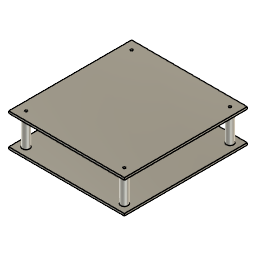
base_colonnine_integrate_dadi_M3_senza_passacavi (Autodesk Fusion 360 design; units mm, degrees)
part number: 2026-07-13-14-09-58-204
part number: 2026-07-13-14-09-58-519
part number: 2026-07-13-14-09-58-558
Autodesk Fusion 360 part; units mm, degrees
sketch "Schizzo1" plane through (0, 0, 0) normal (0, 0, 1) x (1, 0, 0) in component "01_Piano_inferiore_con_colonnine_M3"
  line L0 (-80, -85) -> (80, -85)
  line L1 (80, -85) -> (80, 85)
  line L2 (80, 85) -> (-80, 85)
  line L3 (-80, 85) -> (-80, -85)
extrude "Estrusione_Piano_inferiore" add sketch "Schizzo1" along normal blind 3 makes body 1 in component "01_Piano_inferiore_con_colonnine_M3"
ref_plane "Piano di lavoro1" through (0, 0, 43) normal (0, 0, 1) x (1, 0, 0) in component "02_Piano_superiore"
sketch "Schizzo1 (2)" plane through (0, 0, 43) normal (0, 0, 1) x (1, 0, 0) in component "02_Piano_superiore"
  line L0 (-80, -85) -> (80, -85)
  line L1 (80, -85) -> (80, 85)
  line L2 (80, 85) -> (-80, 85)
  line L3 (-80, 85) -> (-80, -85)
extrude "Estrusione_Piano_superiore" add sketch "Schizzo1 (2)" along normal blind 3 separate body makes body 2 in component "02_Piano_superiore"
ref_plane "Piano di lavoro1" through (0, 0, 3) normal (0, 0, 1) x (1, 0, 0) in component "01_Piano_inferiore_con_colonnine_M3"
ref_plane "Piano di lavoro2" through (0, 0, 40.4) normal (0, 0, 1) x (1, 0, 0) in component "01_Piano_inferiore_con_colonnine_M3"
sketch "Schizzo2" plane through (0, 0, 43) normal (0, 0, 1) x (1, 0, 0) in component "02_Piano_superiore"
  circle A0 centre (-68, -73) radius 1.6
extrude "Foro_M3_superiore_01" cut sketch "Schizzo2" along normal blind 3 bodies 2 in component "02_Piano_superiore"
sketch "Schizzo2 (2)" plane through (0, 0, 3) normal (0, 0, 1) x (1, 0, 0) in component "01_Piano_inferiore_con_colonnine_M3"
  circle A0 centre (-68, -73) radius 5
extrude "Estrusione_Colonnina_M3_01" add sketch "Schizzo2 (2)" along normal blind 40 bodies 1 in component "01_Piano_inferiore_con_colonnine_M3"
sketch "Schizzo3" plane through (0, 0, 0) normal (0, 0, 1) x (1, 0, 0) in component "01_Piano_inferiore_con_colonnine_M3"
  circle A0 centre (-68, -73) radius 1.6
extrude "Foro_passante_M3_colonnina_01" cut sketch "Schizzo3" along normal blind 43 bodies 1 in component "01_Piano_inferiore_con_colonnine_M3"
sketch "Schizzo4" plane through (0, 0, 40.4) normal (0, 0, 1) x (1, 0, 0) in component "01_Piano_inferiore_con_colonnine_M3"
  line L0 (-65.1, -71.3257) -> (-68, -69.6514)
  line L1 (-68, -69.6514) -> (-70.9, -71.3257)
  line L2 (-70.9, -71.3257) -> (-70.9, -74.6743)
  line L3 (-70.9, -74.6743) -> (-68, -76.3486)
  line L4 (-68, -76.3486) -> (-65.1, -74.6743)
  line L5 (-65.1, -74.6743) -> (-65.1, -71.3257)
extrude "Sede_dado_M3_01" cut sketch "Schizzo4" along normal blind 2.6 bodies 1 in component "01_Piano_inferiore_con_colonnine_M3"
sketch "Schizzo3 (2)" plane through (0, 0, 43) normal (0, 0, 1) x (1, 0, 0) in component "02_Piano_superiore"
  circle A0 centre (68, -73) radius 1.6
extrude "Foro_M3_superiore_02" cut sketch "Schizzo3 (2)" along normal blind 3 bodies 2 in component "02_Piano_superiore"
sketch "Schizzo5" plane through (0, 0, 3) normal (0, 0, 1) x (1, 0, 0) in component "01_Piano_inferiore_con_colonnine_M3"
  circle A0 centre (68, -73) radius 5
extrude "Estrusione_Colonnina_M3_02" add sketch "Schizzo5" along normal blind 40 bodies 1 in component "01_Piano_inferiore_con_colonnine_M3"
sketch "Schizzo6" plane through (0, 0, 0) normal (0, 0, 1) x (1, 0, 0) in component "01_Piano_inferiore_con_colonnine_M3"
  circle A0 centre (68, -73) radius 1.6
extrude "Foro_passante_M3_colonnina_02" cut sketch "Schizzo6" along normal blind 43 bodies 1 in component "01_Piano_inferiore_con_colonnine_M3"
sketch "Schizzo7" plane through (0, 0, 40.4) normal (0, 0, 1) x (1, 0, 0) in component "01_Piano_inferiore_con_colonnine_M3"
  line L0 (70.9, -71.3257) -> (68, -69.6514)
  line L1 (68, -69.6514) -> (65.1, -71.3257)
  line L2 (65.1, -71.3257) -> (65.1, -74.6743)
  line L3 (65.1, -74.6743) -> (68, -76.3486)
  line L4 (68, -76.3486) -> (70.9, -74.6743)
  line L5 (70.9, -74.6743) -> (70.9, -71.3257)
extrude "Sede_dado_M3_02" cut sketch "Schizzo7" along normal blind 2.6 bodies 1 in component "01_Piano_inferiore_con_colonnine_M3"
sketch "Schizzo4 (2)" plane through (0, 0, 43) normal (0, 0, 1) x (1, 0, 0) in component "02_Piano_superiore"
  circle A0 centre (68, 73) radius 1.6
extrude "Foro_M3_superiore_03" cut sketch "Schizzo4 (2)" along normal blind 3 bodies 2 in component "02_Piano_superiore"
sketch "Schizzo8" plane through (0, 0, 3) normal (0, 0, 1) x (1, 0, 0) in component "01_Piano_inferiore_con_colonnine_M3"
  circle A0 centre (68, 73) radius 5
extrude "Estrusione_Colonnina_M3_03" add sketch "Schizzo8" along normal blind 40 bodies 1 in component "01_Piano_inferiore_con_colonnine_M3"
sketch "Schizzo9" plane through (0, 0, 0) normal (0, 0, 1) x (1, 0, 0) in component "01_Piano_inferiore_con_colonnine_M3"
  circle A0 centre (68, 73) radius 1.6
extrude "Foro_passante_M3_colonnina_03" cut sketch "Schizzo9" along normal blind 43 bodies 1 in component "01_Piano_inferiore_con_colonnine_M3"
sketch "Schizzo10" plane through (0, 0, 40.4) normal (0, 0, 1) x (1, 0, 0) in component "01_Piano_inferiore_con_colonnine_M3"
  line L0 (70.9, 74.6743) -> (68, 76.3486)
  line L1 (68, 76.3486) -> (65.1, 74.6743)
  line L2 (65.1, 74.6743) -> (65.1, 71.3257)
  line L3 (65.1, 71.3257) -> (68, 69.6514)
  line L4 (68, 69.6514) -> (70.9, 71.3257)
  line L5 (70.9, 71.3257) -> (70.9, 74.6743)
extrude "Sede_dado_M3_03" cut sketch "Schizzo10" along normal blind 2.6 bodies 1 in component "01_Piano_inferiore_con_colonnine_M3"
sketch "Schizzo5 (2)" plane through (0, 0, 43) normal (0, 0, 1) x (1, 0, 0) in component "02_Piano_superiore"
  circle A0 centre (-68, 73) radius 1.6
extrude "Foro_M3_superiore_04" cut sketch "Schizzo5 (2)" along normal blind 3 bodies 2 in component "02_Piano_superiore"
sketch "Schizzo11" plane through (0, 0, 3) normal (0, 0, 1) x (1, 0, 0) in component "01_Piano_inferiore_con_colonnine_M3"
  circle A0 centre (-68, 73) radius 5
extrude "Estrusione_Colonnina_M3_04" add sketch "Schizzo11" along normal blind 40 bodies 1 in component "01_Piano_inferiore_con_colonnine_M3"
sketch "Schizzo12" plane through (0, 0, 0) normal (0, 0, 1) x (1, 0, 0) in component "01_Piano_inferiore_con_colonnine_M3"
  circle A0 centre (-68, 73) radius 1.6
extrude "Foro_passante_M3_colonnina_04" cut sketch "Schizzo12" along normal blind 43 bodies 1 in component "01_Piano_inferiore_con_colonnine_M3"
sketch "Schizzo13" plane through (0, 0, 40.4) normal (0, 0, 1) x (1, 0, 0) in component "01_Piano_inferiore_con_colonnine_M3"
  line L0 (-65.1, 74.6743) -> (-68, 76.3486)
  line L1 (-68, 76.3486) -> (-70.9, 74.6743)
  line L2 (-70.9, 74.6743) -> (-70.9, 71.3257)
  line L3 (-70.9, 71.3257) -> (-68, 69.6514)
  line L4 (-68, 69.6514) -> (-65.1, 71.3257)
  line L5 (-65.1, 71.3257) -> (-65.1, 74.6743)
extrude "Sede_dado_M3_04" cut sketch "Schizzo13" along normal blind 2.6 bodies 1 in component "01_Piano_inferiore_con_colonnine_M3"
component "01_Piano_inferiore_con_colonnine_M3" placed x (1, 0, 0) y (0, 1, 0) z (0, 0, 1) at (0, 0, 0)
component "02_Piano_superiore" placed x (1, 0, 0) y (0, 1, 0) z (0, 0, 1) at (0, 0, 0)
equation "piano_inf_lunghezza = 170.0 mm" comment "Piano inferiore"
equation "piano_inf_larghezza = 160.0 mm" comment "Piano inferiore"
equation "piano_inf_spessore = 3.0 mm" comment "Piano inferiore"
equation "d4 = piano_inf_spessore"
equation "distanza_piani = 40.0 mm" comment "Luce libera fra i piani"
equation "piano_sup_lunghezza = 170.0 mm" comment "Piano superiore"
equation "piano_sup_larghezza = 160.0 mm" comment "Piano superiore"
equation "piano_sup_spessore = 3.0 mm" comment "Piano superiore"
equation "colonnina_diametro = 10.0 mm" comment "Colonnine base"
equation "foro_vite_M3 = 3.2 mm" comment "Gioco vite M3"
equation "colonnina_offset_bordo = 12.0 mm" comment "Centro colonnina dal bordo"
equation "dado_M3_chiave = 5.8 mm" comment "Sede esagonale dado M3"
equation "dado_M3_profondita = 2.6 mm" comment "Profondita sede dado M3"
equation "d15 = piano_inf_spessore + distanza_piani"
equation "d16 = piano_sup_spessore"
equation "d18 = piano_inf_spessore"
equation "d19 = piano_inf_spessore + distanza_piani - dado_M3_profondita"
equation "d20 = piano_sup_spessore"
equation "d22 = distanza_piani"
equation "d24 = piano_inf_spessore + distanza_piani"
equation "d26 = dado_M3_profondita"
equation "d28 = piano_sup_spessore"
equation "d30 = distanza_piani"
equation "d32 = piano_inf_spessore + distanza_piani"
equation "d34 = dado_M3_profondita"
equation "d36 = piano_sup_spessore"
equation "d38 = distanza_piani"
equation "d40 = piano_inf_spessore + distanza_piani"
equation "d42 = dado_M3_profondita"
equation "d44 = piano_sup_spessore"
equation "d46 = distanza_piani"
equation "d48 = piano_inf_spessore + distanza_piani"
equation "d50 = dado_M3_profondita"
named bodies: "Piano_inferiore_con_colonnine_M3", "Piano_superiore"
